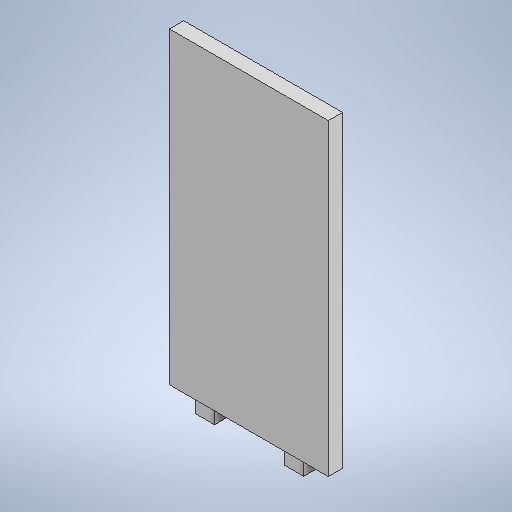
# Autodesk Inventor part: carcasa_piezaLateral_ruedas
Saved by Autodesk Inventor 2025.3 (Build 293356030, 356C)
## iProperties
Created: 2025-09-08
Part Number: carcasa_piezaLateral_ruedas
Material: Generic
Document SubType Name: Modeling
Designer: brene
Density: 1 g/cm^3
Appearance: Default
Author: brene
Autodesk Inventor part; units mm, degrees
ref_plane "YZ Plane" through (0, 0, 0) normal (1, 0, 0) x (0, 1, 0)
ref_plane "XZ Plane" through (0, 0, 0) normal (0, 1, 0) x (-1, 0, 0)
ref_plane "XY Plane" through (0, 0, 0) normal (0, 0, 1) x (1, 0, 0)
sketch "Sketch1" plane through (0, 0, 0) normal (0, 0, 1) x (1, 0, 0)
  line L0 (0, 0) -> (33.5, 0)
  line L1 (33.5, 0) -> (33.5, 65)
  line L2 (33.5, 65) -> (0, 65)
  line L3 (0, 65) -> (0, 0)
  dimension "d0" = 33.5
  dimension "d1" = 65
  dimension "d2" = 33.5
  constraints: 8 end point, 2 perpendicular, 1 horizontal
  measures "d0" distance of L0.start L0.end
  measures "d1" distance of L0.end L1.end
  measures "d2" distance of L1.end L2.end
extrude "Extrusion1" add sketch "Sketch1" along normal blind 3
sketch "Sketch2" plane through (0, 0, 0) normal (0, -1, 0) x (1, 0, 0)
  point P0 (0, 0)
sketch "Sketch3" plane through (0, 0, 0) normal (0, -1, 0) x (1, 0, 0)
  line L0 (0, 0) -> (0, 3) projected
  line L1 (0, 1.5) -> (33.5, 1.5)
  line L2 (33.5, 0) -> (33.5, 3) projected
  line L3 (16.75, 1.5) -> (9.347, 1.5)
  line L4 (9.347, 1.5) -> (9.347, 2.85)
  line L5 (9.347, 2.85) -> (5.347, 2.85)
  line L6 (5.347, 2.85) -> (5.347, 0.15)
  line L7 (5.347, 0.15) -> (9.347, 0.15)
  line L8 (9.347, 0.15) -> (9.347, 1.5)
  line L9 (16.75, 1.5) -> (24.153, 1.5)
  line L10 (24.153, 1.5) -> (24.153, 2.85)
  line L11 (24.153, 2.85) -> (28.153, 2.85)
  line L12 (28.153, 2.85) -> (28.153, 0.15)
  line L13 (28.153, 0.15) -> (24.153, 0.15)
  line L14 (24.153, 0.15) -> (24.153, 1.5)
  dimension "d5" = 7.403
  dimension "d6" = 1.35
  dimension "d7" = 4
  dimension "d9" = 2.7
  dimension "d10" = 4
  dimension "d11" = 7.403
  dimension "d12" = 1.35
  dimension "d13" = 4
  dimension "d14" = 2.7
  dimension "d15" = 4
  constraints: 26 end point, 5 perpendicular, 4 point on line, 3 midpoint, 1 vertical
  measures "d5" distance of L3.start L3.end
  measures "d6" distance of L3.end L4.end
  measures "d7" distance of L4.end L5.end
  measures "d9" distance of L5.end L6.end
  measures "d10" distance of L6.end L7.end
  measures "d11" distance of L3.start L9.end
  measures "d12" distance of L9.end L10.end
  measures "d13" distance of L10.end L11.end
  measures "d14" distance of L11.end L12.end
  measures "d15" distance of L12.end L13.end
extrude "Extrusion2" add sketch "Sketch3" along normal blind 2.7
body "Solid1"
